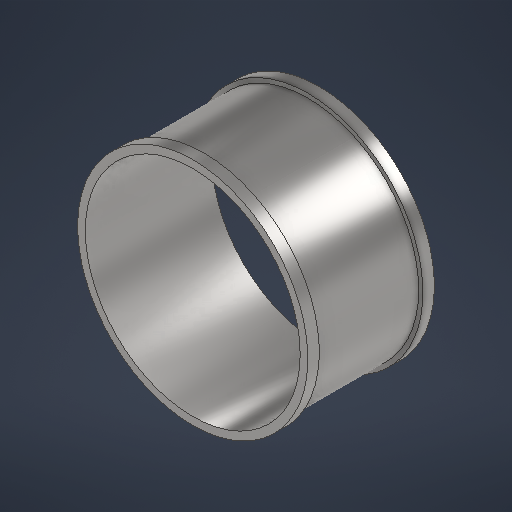
# Autodesk Inventor part: DiscoCorpoTurbina2
Saved by Autodesk Inventor 2026.2 (Build 302298010, 298A)
## iProperties
Created: 2026-04-30
Part Number: DiscoCorpoTurbina2
Material: Steel, Alloy
Document SubType Name: Modeling
Designer: Yan
Density: 7.73 g/cm^3
Appearance: Semi-Polished
Author: Yan
Autodesk Inventor part; units mm, degrees
ref_plane "YZ Plane" through (0, 0, 0) normal (1, 0, 0) x (0, 1, 0)
ref_plane "XZ Plane" through (0, 0, 0) normal (0, 1, 0) x (-1, 0, 0)
ref_plane "XY Plane" through (0, 0, 0) normal (0, 0, 1) x (1, 0, 0)
sketch "Sketch1" plane through (0, 0, 0) normal (1, 0, 0) x (0, 1, 0)
  line L0 (0, 0) -> (0, -445)
  line L1 (0, -445) -> (378, -445)
  line L2 (378, -445) -> (378, 0)
  line L3 (378, 0) -> (0, 0)
  line L4 (378, -445) -> (405, -445)
  line L5 (405, -445) -> (405, -405)
  line L6 (405, -405) -> (390, -405)
  line L7 (390, -405) -> (390, -40)
  line L8 (390, -40) -> (405, -40)
  line L9 (405, -40) -> (405, 0)
  line L10 (405, 0) -> (378, 0)
  dimension "d0" = 756
  dimension "d1" = 445
  dimension "d2" = 40
  dimension "d3" = 40
  dimension "d4" = 780
  dimension "d5" = 810
  constraints: 22 end point, 8 perpendicular, 2 point on line, 1 horizontal, 1 vertical
  measures "d0" diameter of L2 L0
  measures "d1" distance of L0.start L0.end
  measures "d2" distance of L8.end L9.end
  measures "d3" distance of L4.end L5.end
  measures "d4" diameter of L7 L0
  measures "d5" diameter of L9 L0
revolve "Revolution1" add sketch "Sketch1" angle 360 about axis through (0, 0, 0) along (0, 0, -1) contours L10 L9 L8 L7 L6 L5 L4 L2
body "Solid1"
